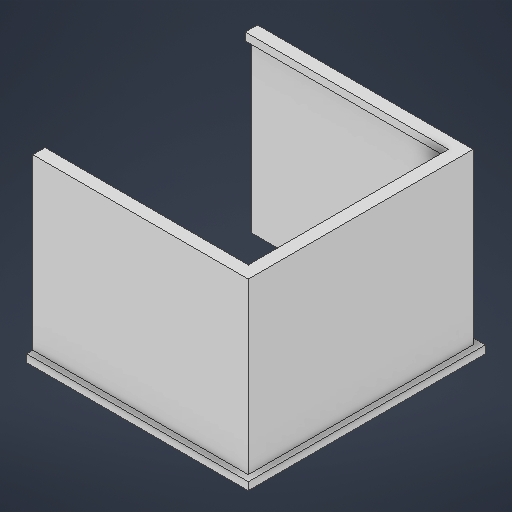
# Autodesk Inventor part: Galvo Housing-01
Saved by Autodesk Inventor 2025 (Build 290162000, 162)
## iProperties
Created: 2024-06-12
Part Number: Galvo Housing-01
Material: Generic
Document SubType Name: Modeling
Designer: mayhe
Density: 1 g/cm^3
Appearance: Default
Author: mayhe
Autodesk Inventor part; units mm, degrees
ref_plane "YZ Plane" through (0, 0, 0) normal (1, 0, 0) x (0, 1, 0)
ref_plane "XZ Plane" through (0, 0, 0) normal (0, 1, 0) x (-1, 0, 0)
ref_plane "XY Plane" through (0, 0, 0) normal (0, 0, 1) x (1, 0, 0)
sketch "Sketch4" plane through (0, 0, 0) normal (0, 1, 0) x (-1, 0, 0)
  line L0 (-70, 73) -> (70, 73)
  line L1 (70, -73) -> (-70, -73)
  line L2 (-70, -73) -> (-70, 73)
  line L3 (-66, -69) -> (70, -69)
  line L4 (70, 69) -> (-66, 69)
  line L5 (-66, 69) -> (-66, -69)
  line L6 (70, 73) -> (70, 69)
  line L7 (70, -69) -> (70, -73)
  point P0 (0, 0)
  dimension "Housing_Length" = 140
  dimension "Housing_Width" = 146
  dimension "d15" = 4
  constraints: 16 end point, 4 parallel, 2 perpendicular, 1 horizontal
  measures "Housing_Length" distance of L1.start L1.end
  measures "Housing_Width" distance of L0.end L1.start
  measures "d15" distance between parallel lines of L1 L3
extrude "Extrusion4" add sketch "Sketch4" along normal blind 115
sketch "Sketch6" plane through (0, 115, 0) normal (0, 1, 0) x (1, 0, 0)
  line L0 (70, 73) -> (-70, 73) projected
  line L1 (-70, -69) -> (-70, -73) projected
  line L2 (70, 73) -> (-70, 73)
  line L3 (-70, 73) -> (-70, -73)
  line L4 (-70, -73) -> (70, -73)
  line L5 (70, -73) -> (70, 73)
  line L6 (62, -65) -> (-70, -65)
  line L7 (-70, 65) -> (62, 65)
  line L8 (62, 65) -> (62, -65)
  point P0 (0, 0)
  dimension "Lip_Width" = 8
  constraints: 14 end point, 3 parallel, 2 point on line, 1 horizontal, 1 perpendicular
  measures "Lip_Width" distance between parallel lines of L4 L6
extrude "Extrusion5" add sketch "Sketch6" against normal blind 5 contours L5 L4 L1 L3 L6 L8 L7 L0
sketch "Sketch7" plane through (0, 0, 0) normal (0, -1, 0) x (1, 0, 0)
  line L0 (-70, -73) -> (-70, -69) projected
  line L1 (-70, 73) -> (70, 73) projected
  line L2 (-70, -73) -> (70, -73)
  line L3 (70, -73) -> (70, 73)
  line L4 (70, 73) -> (-70, 73)
  line L5 (-70, 77) -> (-70, -73)
  line L6 (74, 77) -> (74, -77)
  line L7 (74, -77) -> (-70, -77)
  line L8 (-70, 77) -> (74, 77)
  line L9 (-70, -73) -> (-70, -77)
  point P0 (0, 0)
  dimension "d23" = 4
  constraints: 16 end point, 3 parallel, 3 perpendicular, 1 horizontal, 1 point on line
  measures "d23" distance between parallel lines of L3 L6
extrude "Extrusion6" add sketch "Sketch7" against normal blind 5 contours L2 L3 L1 L5 L8 L6 L7 L9
body "Solid2"
